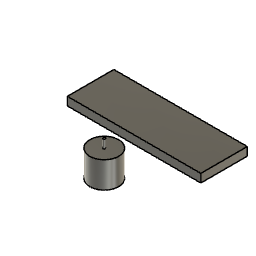
assembly v4 (Autodesk Fusion 360 design; units mm, degrees)
Autodesk Fusion 360 part; units mm, degrees
sketch "Sketch1" plane through (0, 0, 0) normal (0, 0, 1) x (1, 0, 0)
  circle A0 centre (0, 0) radius 17.275
  dimension "d1" = 34.55
  constraint coincident A0.centre origin
  measures "d1" diameter of A0
extrude "Extrude1" add sketch "Sketch1" along normal blind 31.55 makes body 1
sketch "Sketch2" plane through (0, 0, 31.55) normal (0, 0, 1) x (-1, 0, 0)
  circle A0 centre (0, 0) radius 17.275
  circle A1 centre (0, 0) radius 1.495
  dimension "d4" = 2.99
  constraint concentric A0 A1
  measures "d4" diameter of A1
extrude "Extrude2" add sketch "Sketch2" along normal blind 10 contours A1 bodies 1
sketch "Sketch3" plane through (0, 0, 0) normal (0, 0, 1) x (1, 0, 0)
  line L0 (62.7346, 53.1278) -> (-97.3754, 53.1278)
  line L1 (-97.3754, 53.1278) -> (-97.3754, 108.8778)
  line L2 (-97.3754, 108.8778) -> (62.7346, 108.8778)
  line L3 (62.7346, 108.8778) -> (62.7346, 53.1278)
  dimension "d7" = 160.11
  dimension "d8" = 55.75
  constraint horizontal L0
  constraint vertical L1
  constraint horizontal L2
  constraint vertical L3
  measures "d7" distance of L0.start L0.end
  measures "d8" distance of L0.start L2.end
extrude "Extrude3" add sketch "Sketch3" along normal blind 10 separate body makes body 2
